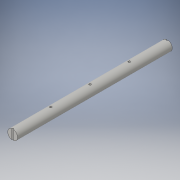
# Autodesk Inventor part: Straw
Saved by Autodesk Inventor 2016 (Build 200138000, 138)
## iProperties
Created: 2017-04-26
Part Number: Straw
Material: Generic
Document SubType Name: Modeling
Designer: wtse3759
Density: 1 g/cm^3
Appearance: Default
Author: wtse3759
Autodesk Inventor part; units mm, degrees
ref_plane "YZ Plane" through (0, 0, 0) normal (1, 0, 0) x (0, 1, 0)
ref_plane "XZ Plane" through (0, 0, 0) normal (0, 1, 0) x (-1, 0, 0)
ref_plane "XY Plane" through (0, 0, 0) normal (0, 0, 1) x (1, 0, 0)
sketch "Sketch1" plane through (0, 0, 0) normal (0, 0, 1) x (1, 0, 0)
  circle A0 centre (0, 0) radius 6.35
  dimension "d0" = 12.7
  constraints: 1 centre point, 1 coincident
  measures "d0" diameter of A0
extrude "Extrusion1" add sketch "Sketch1" along normal blind 203.2
sketch "Sketch4" plane through (0, 0, 0) normal (0, 1, 0) x (-1, 0, 0)
  line L0 (0, 0) -> (0, 1.524)
  line L1 (6.35, 203.2) -> (-6.35, 203.2) projected
  line L2 (0, 203.2) -> (0, 201.676)
  circle A0 centre (0, 201.676) radius 1.27
  circle A1 centre (0, 1.524) radius 1.27
  dimension "d13" = 1.524
  dimension "d15" = 1.524
  dimension "d16" = 2.54
  dimension "d19" = 2.54
  constraints: 4 end point, 2 centre point, 2 coincident, 2 vertical, 1 midpoint
  measures "d13" distance of L0.start L0.end
  measures "d15" distance of L2.start L2.end
  measures "d16" diameter of A0
  measures "d19" diameter of A1
extrude "Extrusion4" cut sketch "Sketch4" along normal mid plane 15.24
sketch "Sketch5" plane through (0, 0, 0) normal (0, 1, 0) x (-1, 0, 0)
  line L0 (0, 1.524) -> (-1.27, 1.524)
  line L1 (-6.35, 0) -> (6.35, 0) projected
  line L2 (-1.27, 0) -> (1.27, 0)
  line L3 (1.27, 1.524) -> (0, 1.524)
  line L4 (1.27, 1.524) -> (6.35, 1.524)
  line L5 (6.35, 0) -> (6.35, 203.2) projected
  line L6 (6.35, 1.524) -> (-6.35, 1.524)
  line L7 (-6.35, 1.524) -> (-6.35, 0)
  line L8 (-6.35, 0) -> (6.35, 0)
  line L9 (6.35, 0) -> (6.35, 1.524)
  line L10 (6.35, 203.2) -> (-6.35, 203.2) projected
  line L11 (-6.35, 203.2) -> (6.35, 203.2)
  line L12 (6.35, 203.2) -> (6.35, 201.676)
  line L13 (6.35, 201.676) -> (-6.35, 201.676)
  line L14 (-6.35, 201.676) -> (-6.35, 203.2)
  point P0 (0, 0)
  dimension "d20" = 1.524
  dimension "d21" = 1.27
  dimension "d26" = 12.7
  dimension "d27" = 1.524
  constraints: 24 end point, 5 equal length, 4 point on line, 3 horizontal, 2 perpendicular
  measures "d20" distance of point (0, 0) L0.start
  measures "d21" distance of L0.start L0.end
  measures "d26" distance of L12.end L13.end
  measures "d27" distance of L11.end L12.end
extrude "Extrusion6" cut sketch "Sketch5" along normal mid plane 25.4
sketch "Sketch6" plane through (0, 0, 0) normal (0, 1, 0) x (-1, 0, 0)
  line L0 (-6.35, 0) -> (-6.35, 50.8)
  line L1 (-6.35, 50.8) -> (0, 50.8)
  line L2 (6.35, 1.524) -> (6.35, 201.676) projected
  circle A0 centre (0, 50.8) radius 1.27
  line L3 (-6.35, 101.6) -> (0, 101.6)
  line L4 (0, 50.8) -> (0, 101.6)
  circle A1 centre (0, 101.6) radius 1.27
  line L5 (0, 101.6) -> (0, 152.4)
  circle A2 centre (0, 152.4) radius 1.27
  line L6 (0, 152.4) -> (0, 203.2)
  point P0 (0, 0)
  dimension "d30" = 50.8
  dimension "d31" = 50.8
  dimension "d33" = 6.35
  dimension "d34" = 2.54
  dimension "d36" = 2.54
  dimension "d37" = 50.8
  dimension "d38" = 2.54
  dimension "d39" = 50.8
  constraints: 12 end point, 3 centre point, 3 coincident, 2 perpendicular, 1 horizontal, 1 point on line, 1 vertical
  measures "d30" distance of L0.start L0.end
  measures "d31" distance of L0.end L3.start
  measures "d33" distance of L0.end L1.end
  measures "d34" diameter of A0
  measures "d36" diameter of A1
  measures "d37" distance of L5.start L5.end
  measures "d38" diameter of A2
  measures "d39" distance of L6.start L6.end
extrude "Extrusion7" cut sketch "Sketch6" along normal mid plane 25.4
body "Solid1"
